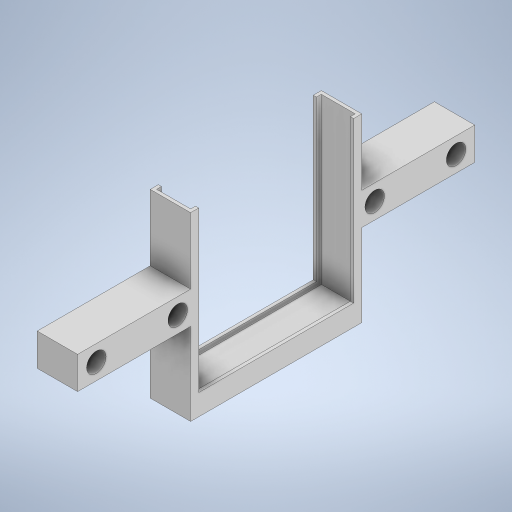
# Autodesk Inventor part: FanPTMounts
Saved by Autodesk Inventor 2024.1 (Build 281209000, 209)
## iProperties
Created: 2024-05-07
Part Number: FanPTMounts
Material: Generic
Document SubType Name: Modeling
Designer: chihs
Density: 1 g/cm^3
Appearance: Default
Author: chihs
Autodesk Inventor part; units mm, degrees
ref_plane "YZ Plane" through (0, 0, 0) normal (1, 0, 0) x (0, 1, 0)
ref_plane "XZ Plane" through (0, 0, 0) normal (0, 1, 0) x (-1, 0, 0)
ref_plane "XY Plane" through (0, 0, 0) normal (0, 0, 1) x (1, 0, 0)
sketch "Sketch1" plane through (0, 0, 0) normal (1, 0, 0) x (0, 1, 0)
  line L0 (0, 0) -> (52, 0)
  line L1 (52, 0) -> (52, -53)
  line L2 (52, -53) -> (0, -53)
  line L3 (0, -53) -> (0, 0)
  line L4 (0, 0) -> (2.5, 0) construction
  line L5 (2.5, 0) -> (2.5, -2.5) construction
  line L6 (52, -53) -> (52, -50.5) construction
  line L7 (52, 0) -> (52, -2.5) construction
  line L8 (2.5, -2.5) -> (52, -2.5)
  line L9 (52, -2.5) -> (52, -50.5)
  line L10 (52, -50.5) -> (2.5, -50.5)
  line L11 (2.5, -50.5) -> (2.5, -2.5)
  dimension "d0" = 53
  dimension "d1" = 52
  dimension "d2" = 2.5
  dimension "d3" = 2.5
  dimension "d4" = 2.5
  dimension "d5" = 2.5
  constraints: 24 end point, 5 parallel, 3 point on line, 2 horizontal, 2 perpendicular
  measures "d0" distance of L0.end L1.end
  measures "d1" distance of L1.end L2.end
  measures "d2" distance of L0.start L4.end
  measures "d3" distance of L4.end L5.end
  measures "d4" distance of L1.end L6.end
  measures "d5" distance of L0.end L7.end
extrude "Extrusion1" add sketch "Sketch1" along normal blind 12.5 contours L0 L1 L8 L11 L10 L2 L3
sketch "Sketch2" plane through (0, 52, -50.5) normal (0, 1, 0) x (1, 0, 0)
  line L0 (12.5, 2.5) -> (12.5, 0) construction
  line L1 (12.5, 2.5) -> (11.5, 2.5) construction
  line L2 (0, 2.5) -> (12.5, 2.5) construction
  line L3 (11.5, 2.5) -> (11.5, 1.5) construction
  line L4 (0, 2.5) -> (1, 2.5) construction
  line L5 (1, 2.5) -> (1, 1.5) construction
  line L6 (0, -50.5) -> (12.5, -50.5) construction
  line L7 (12.5, -50.5) -> (11.5, -50.5) construction
  line L8 (11.5, -50.5) -> (11.5, -49.5) construction
  line L9 (0, -50.5) -> (1, -50.5) construction
  line L10 (1, -50.5) -> (1, -49.5) construction
  line L11 (1, -49.5) -> (11.5, -49.5)
  line L12 (11.5, -49.5) -> (11.5, -48)
  line L13 (11.5, -48) -> (1, -48)
  line L14 (1, -48) -> (1, -49.5)
  line L15 (1, 1.5) -> (11.5, 1.5)
  line L16 (11.5, 1.5) -> (11.5, 0)
  line L17 (11.5, 0) -> (1, 0)
  line L18 (1, 0) -> (1, 1.5)
  dimension "d8" = 1
  dimension "d9" = 1
  dimension "d10" = 1
  dimension "d11" = 1
  dimension "d14" = 1
  dimension "d15" = 1
  dimension "d16" = 1
  dimension "d17" = 1
  dimension "d18" = 1.5
  dimension "d19" = 10.5
  dimension "d20" = 10.5
  dimension "d21" = 1.5
  constraints: 32 end point, 5 perpendicular, 4 parallel, 4 point on line, 2 horizontal, 1 vertical
  measures "d8" distance of L0.start L1.end
  measures "d9" distance of L1.end L3.end
  measures "d10" distance of L2.start L4.end
  measures "d11" distance of L4.end L5.end
  measures "d14" distance of L6.end L7.end
  measures "d15" distance of L7.end L8.end
  measures "d16" distance of L6.start L9.end
  measures "d17" distance of L9.end L10.end
  measures "d18" distance of L11.end L12.end
  measures "d19" distance of L10.end L11.end
  measures "d20" distance of L5.end L15.end
  measures "d21" distance of L17.end L5.end
extrude "Extrusion2" cut sketch "Sketch2" against normal blind 51
sketch "Sketch3" plane through (0, 2.5, -2.5) normal (0, 1, 0) x (1, 0, 0)
  line L0 (0, -2.5) -> (1, -2.5) construction
  line L1 (0, -2.5) -> (12.5, -2.5) construction
  line L2 (0, -2.5) -> (0, -1.5) construction
  line L3 (0, -2.5) -> (0, 50.5) construction
  line L4 (0, -1.5) -> (1, -1.5) construction
  line L5 (1, -1.5) -> (11.5, -1.5)
  line L6 (11.5, -1.5) -> (11.5, 49.5)
  line L7 (11.5, 49.5) -> (1, 49.5)
  line L8 (1, 49.5) -> (1, -1.5)
  dimension "d23" = 1
  dimension "d24" = 1
  dimension "d25" = 10.5
  dimension "d26" = 51
  constraints: 14 end point, 2 parallel, 2 perpendicular, 2 point on line, 1 horizontal
  measures "d23" distance of L0.start L2.end
  measures "d24" distance of L2.end L4.end
  measures "d25" distance of L6.end L7.end
  measures "d26" distance of L7.end L4.end
extrude "Extrusion3" cut sketch "Sketch3" against normal blind 1.5
sketch "Sketch4" plane through (12.5, 0, 0) normal (1, 0, 0) x (0, 0, -1)
  line L0 (53, 52) -> (50.5, 52) construction
  line L1 (53, 52) -> (53, 26.5) construction
  line L2 (53, 26.5) -> (108.8773, 26.5) construction
  line L3 (53, 26.5) -> (53, 31.5) construction
  line L4 (53, 0) -> (53, 52) construction
  line L5 (53, 31.5) -> (88, 31.5)
  line L6 (88, 31.5) -> (88, 21.5)
  line L7 (88, 21.5) -> (53, 21.5)
  line L8 (53, 21.5) -> (53, 31.5)
  line L9 (0, 52) -> (0, 26.5) construction
  line L10 (0, 52) -> (0, 0) construction
  line L11 (0, 26.5) -> (-54.8348, 26.5) construction
  line L12 (0, 26.5) -> (0, 31.5) construction
  line L13 (0, 31.5) -> (-35, 31.5)
  line L14 (-35, 31.5) -> (-35, 21.5)
  line L15 (-35, 21.5) -> (0, 21.5)
  line L16 (0, 21.5) -> (0, 31.5)
  dimension "d29" = 25.5
  dimension "d30" = 5
  dimension "d31" = 10
  dimension "d32" = 35
  dimension "d41" = 25.5
  dimension "d42" = 5
  dimension "d43" = 35
  dimension "d44" = 10
  constraints: 28 end point, 4 parallel, 3 horizontal, 3 perpendicular, 3 point on line, 1 vertical
  measures "d29" distance of L0.start L1.end
  measures "d30" distance of L1.end L3.end
  measures "d31" distance of L5.end L6.end
  measures "d32" distance of L6.end L7.end
  measures "d41" distance of L9.start L9.end
  measures "d42" distance of L9.end L12.end
  measures "d43" distance of L12.end L13.end
  measures "d44" distance of L13.end L14.end
extrude "Extrusion4" add sketch "Sketch4" against normal blind 12.5
sketch "Sketch5" plane through (12.5, 0, 0) normal (1, 0, 0) x (0, 0, -1)
  line L0 (53, 52) -> (50.5, 52) construction
  line L1 (50.5, 52) -> (50.5, 26.5) construction
  line L2 (50.5, 52) -> (50.5, 2.5) construction
  line L3 (50.5, 26.5) -> (53, 26.5) construction
  line L4 (53, 26.5) -> (57, 26.5) construction
  circle A0 centre (57, 26.5) radius 3
  line L5 (57, 26.5) -> (82.2, 26.5) construction
  circle A1 centre (82.2, 26.5) radius 3
  line L6 (0, 52) -> (0, 26.5) construction
  line L7 (0, 26.5) -> (-4, 26.5) construction
  line L8 (-4, 26.5) -> (-29.2, 26.5) construction
  circle A2 centre (-4, 26.5) radius 3
  circle A3 centre (-29.2, 26.5) radius 3
  point P0 (0, 0)
  dimension "d35" = 25.5
  dimension "d36" = 2.5
  dimension "d37" = 6
  dimension "d38" = 4
  dimension "d39" = 25.2
  dimension "d40" = 6
  dimension "d45" = 25.5
  dimension "d46" = 4
  dimension "d47" = 25.2
  dimension "d48" = 6
  dimension "d49" = 6
  constraints: 14 end point, 4 centre point, 4 coincident, 4 horizontal, 2 point on line, 1 vertical
  measures "d35" distance of L0.end L1.end
  measures "d36" distance of L1.end L3.end
  measures "d37" diameter of A0
  measures "d38" distance of L3.end L4.end
  measures "d39" distance of L5.start L5.end
  measures "d40" diameter of A1
  measures "d45" distance of L6.start L6.end
  measures "d46" distance of L6.end L7.end
  measures "d47" distance of L7.end L8.end
  measures "d48" diameter of A2
  measures "d49" diameter of A3
extrude "Extrusion5" cut sketch "Sketch5" against normal blind 12.5
sketch "Sketch6" plane through (0, 0, -53) normal (0, -1, 0) x (1, 0, 0)
  line L0 (12.5, 53) -> (0, 53)
  line L1 (0, 53) -> (0, 0)
  line L2 (0, 0) -> (12.5, 0)
  line L3 (12.5, 0) -> (12.5, 53)
  line L4 (12.5, 53) -> (12.5, 0) projected
  dimension "d54" = 0
  constraints: 8 end point, 2 parallel, 1 horizontal, 1 perpendicular
  measures "d54" distance between parallel lines of L4 L3
extrude "Extrusion6" add sketch "Sketch6" along normal blind 4
sketch "Sketch7" plane through (0, -4, -53) normal (0, -1, 0) x (1, 0, 0)
  line L0 (12.5, 53) -> (0, 53) construction
  line L1 (6.25, 53) -> (6.25, 26.5) construction
  circle A0 centre (6.25, 26.5) radius 0.5
  dimension "d55" = 26.5
  dimension "d56" = 1
  constraints: 2 end point, 1 centre point, 1 coincident, 1 midpoint, 1 vertical
  measures "d55" distance of L1.start L1.end
  measures "d56" diameter of A0
extrude "Extrusion7" cut sketch "Sketch7" against normal blind 1
equation "\"d0\" = lfan + 2 * thickness"
equation "\"d1\" = lfan + thickness"
equation "\"d2\" = fanclip"
equation "\"d3\" = fanclip"
equation "\"d4\" = fanclip"
equation "\"d5\" = fanclip"
equation "\"d6\" = tfan + 2 * thickness"
equation "\"d8\" = thickness"
equation "\"d9\" = thickness"
equation "\"d10\" = thickness"
equation "\"d11\" = thickness"
equation "\"d14\" = thickness"
equation "\"d15\" = thickness"
equation "\"d16\" = thickness"
equation "\"d17\" = thickness"
equation "\"d18\" = fanclip - thickness"
equation "\"d19\" = tfan"
equation "\"d20\" = tfan"
equation "\"d21\" = fanclip - thickness"
equation "\"d12\" = lfan"
equation "\"d23\" = thickness"
equation "\"d24\" = thickness"
equation "\"d25\" = tfan"
equation "\"d26\" = lfan"
equation "\"d27\" = fanclip - thickness"
equation "\"d29\" = 0.5 * lfan"
equation "\"d30\" = 0.5 * twing"
equation "\"d31\" = twing"
equation "\"d32\" = lwing"
equation "\"d41\" = 0.5 * lfan"
equation "\"d42\" = 0.5 * twing"
equation "\"d43\" = lwing"
equation "\"d44\" = twing"
equation "\"d33\" = tfan + 2 * thickness"
equation "\"d35\" = 0.5 * lfan"
equation "\"d36\" = fanclip"
equation "\"d37\" = dPhoto"
equation "\"d38\" = gapto1"
equation "\"d39\" = gapto2"
equation "\"d40\" = dPhoto"
equation "\"d45\" = 0.5 * lfan"
equation "\"d46\" = gapto1"
equation "\"d47\" = gapto2"
equation "\"d48\" = dPhoto"
equation "\"d49\" = dPhoto"
equation "\"d50\" = tfan + 2 * thickness"
equation "\"d52\" = 4 * thickness"
equation "\"d55\" = 0.5 * lfan + thickness"
equation "\"d57\" = thickness"
equation "\"lfan\" = 51"
equation "\"tfan\" = 10.5"
equation "\"thickness\" = 1"
equation "\"fanclip\" = 2.5"
equation "\"twing\" = 10"
equation "\"lwing\" = 35"
equation "\"dPhoto\" = 6"
equation "\"gapto1\" = 4"
equation "\"gapto2\" = 25.2"
body "Solid1"
